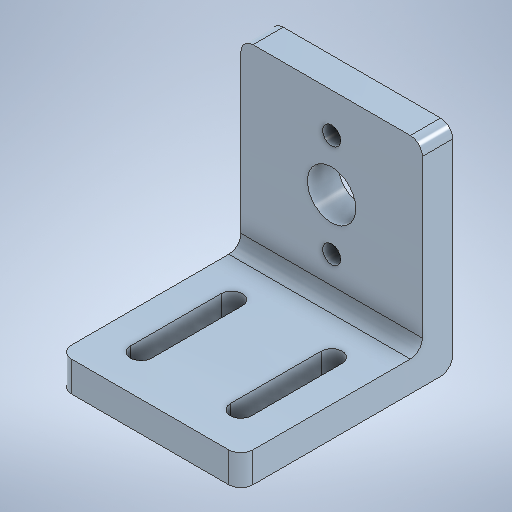
# Autodesk Inventor part: soporte_motor
Saved by Autodesk Inventor 2026 (Build 300175050, 175E)
## iProperties
Created: 2025-08-26
Part Number: soporte_motor
Material: Genérico
Document SubType Name: Modeling
Designer: piero
Density: 1 g/cm^3
Appearance: Valor por defecto
Author: piero
Autodesk Inventor part; units mm, degrees
ref_plane "YZ Plane" through (0, 0, 0) normal (1, 0, 0) x (0, 1, 0)
ref_plane "XZ Plane" through (0, 0, 0) normal (0, 1, 0) x (-1, 0, 0)
ref_plane "XY Plane" through (0, 0, 0) normal (0, 0, 1) x (1, 0, 0)
sketch "Boceto1" plane through (0, 0, 0) normal (0, 0, 1) x (1, 0, 0)
  line L0 (0, 0) -> (30, 0)
  line L1 (30, 0) -> (30, 30)
  line L2 (30, 30) -> (0, 30)
  line L3 (0, 30) -> (0, 0)
  circle A0 centre (15, 15) radius 4
  circle A1 centre (15, 23.5) radius 1.5
  circle A2 centre (15, 6.5) radius 1.5
  dimension "d0" = 30
  dimension "d1" = 30
  dimension "d2" = 8
  dimension "d3" = 3
  dimension "d4" = 3
  dimension "d5" = 8.5
  dimension "d6" = 8.5
  dimension "d7" = 6.5
  constraints: 8 end point, 3 centre point, 2 parallel, 1 horizontal, 1 perpendicular
  measures "d0" distance of L2.end L1.end
  measures "d1" distance of L1.end L0.end
  measures "d2" diameter of A0
  measures "d3" diameter of A1
  measures "d4" diameter of A2
  measures "d5" distance of A0.centre A1.centre
  measures "d6" distance of A0.centre A2.centre
  measures "d7" distance from line of L2 A1.centre
extrude "Extrusión1" add sketch "Boceto1" along normal blind 5
sketch "Boceto2" plane through (0, 0, 0) normal (0, 0, -1) x (-1, 0, 0)
  line L0 (-30, 0) -> (-30, 30) projected
  line L1 (-30, 0) -> (0, 0)
  line L2 (0, 0) -> (0, -5)
  line L3 (0, -5) -> (-30, -5)
  line L4 (-30, -5) -> (-30, 0)
  dimension "d10" = 5
  constraints: 8 end point, 2 parallel, 1 horizontal, 1 perpendicular
  measures "d10" distance of L1.end L2.end
extrude "Extrusión2" add sketch "Boceto2" against normal blind 35
sketch "Boceto3" plane through (0, 0, 5) normal (0, 1, 0) x (1, 0, 0)
  line L0 (6.75, -8.25) -> (6.75, -23.25) construction
  line L1 (5, -8.25) -> (5, -23.25)
  line L2 (8.5, -23.25) -> (8.5, -8.25)
  arc A0 (8.5, -8.25) -> (5, -8.25) centre (6.75, -8.25) ccw
  arc A1 (5, -23.25) -> (8.5, -23.25) centre (6.75, -23.25) ccw
  line L3 (23.25, -8.25) -> (23.25, -23.25) construction
  line L4 (21.5, -8.25) -> (21.5, -23.25)
  line L5 (25, -23.25) -> (25, -8.25)
  arc A2 (25, -8.25) -> (21.5, -8.25) centre (23.25, -8.25) ccw
  arc A3 (21.5, -23.25) -> (25, -23.25) centre (23.25, -23.25) ccw
  line L6 (0, 0) -> (0, -30) projected
  line L7 (30, 0) -> (30, -30) projected
  line L8 (30, -30) -> (0, -30) projected
  point P0 (0, 5)
  point P1 (6.75, -15.75)
  point P2 (23.25, -15.75)
  point P3 (6.75, -25)
  dimension "d13" = 3.5
  dimension "d14" = 3.5
  dimension "d15" = 15
  dimension "d16" = 15
  dimension "d17" = 5
  dimension "d18" = 5
  dimension "d19" = 0
  dimension "d20" = 5
  constraints: 16 end point, 9 point on circle, 8 tangent, 4 centre point, 2 midpoint, 2 parallel, 2 vertical
  measures "d13" diameter of A1
  measures "d14" diameter of A3
  measures "d15" distance of L2.start L2.end
  measures "d16" distance of L4.start L4.end
  measures "d17" distance between parallel lines of L6 L1
  measures "d18" distance between parallel lines of L7 L5
  measures "d19" vertical distance of L4.start L2.end
  measures "d20" distance from line of L8 point (6.75, -25)
extrude "Extrusión3" cut sketch "Boceto3" against normal blind 5
fillet "Empalme1" radius 2 1 edges at (15, -5, 0)
fillet "Empalme2" radius 2 5 edges at (0, -2.5, 35) (30, -2.5, 35) (30, 30, 2.5) (0, 30, 2.5) (15, 0, 5)
